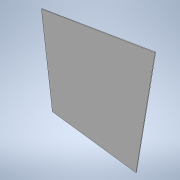
# Autodesk Inventor part: TableTop
Saved by Autodesk Inventor 2022 (Build 260153000, 153)
## iProperties
Created: 2022-01-15
Part Number: TableTop
Material: Generic
Document SubType Name: Modeling
Designer: dangl
Density: 1 g/cm^3
Appearance: Default
Author: dangl
Autodesk Inventor part; units mm, degrees
ref_plane "YZ Plane" through (0, 0, 0) normal (1, 0, 0) x (0, 1, 0)
ref_plane "XZ Plane" through (0, 0, 0) normal (0, 1, 0) x (-1, 0, 0)
ref_plane "XY Plane" through (0, 0, 0) normal (0, 0, 1) x (1, 0, 0)
sketch "Sketch1" plane through (0, 0, 0) normal (0, 0, 1) x (1, 0, 0)
  line L0 (457.2, -457.2) -> (-457.2, -457.2)
  line L1 (-457.2, -457.2) -> (-457.2, 457.2)
  line L2 (-457.2, 457.2) -> (457.2, 457.2)
  line L3 (457.2, 457.2) -> (457.2, -457.2)
  point P0 (0, 0)
  dimension "d0" = 914.4
  dimension "d1" = 914.4
  dimension "d2" = 457.2
  dimension "d3" = 457.2
  constraints: 8 end point, 2 parallel, 1 horizontal, 1 perpendicular
  measures "d0" distance of L0.start L0.end
  measures "d1" distance of L0.end L1.end
  measures "d2" distance from line of point (0, 0) L0
  measures "d3" distance from line of point (0, 0) L3
extrude "Extrusion1" add sketch "Sketch1" against normal blind 19.05 draft -55
extrude "Extrusion2" add sketch "Sketch1" along normal blind 6.35
equation "\"d1\" = d0"
equation "\"d2\" = 0.5 * d0"
equation "\"d3\" = d2"
body "Solid1"
